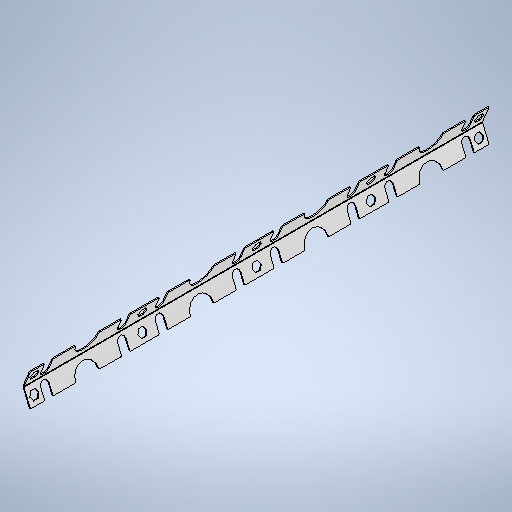
# Autodesk Inventor part: DMF 01 17 опора крышки v2.1
Saved by Autodesk Inventor 2026.2 (Build 302298010, 298A)
## iProperties
Created: 2024-04-30
Part Number: DMF 01 17 опора крышки v2.1
Material: Stainless Steel AISI 304
Document SubType Name: Sheet Metal
Designer: pokla
Density: 8 g/cm^3
Appearance: Chrome - Satin
Sheet Metal Rule: Default
Flat Pattern Width: 7.47819 cm
Flat Pattern Length: 98.3 cm
Flat Pattern Area: 735.107 cm^2
Sheet Metal Width: 74,782 mm
Sheet Metal Length: 983,000 mm
Sheet Metal Area: 73510,654 mm^2
Stock Number: Барабан_Полка_Крышки
Author: pokla
Autodesk Inventor part; units mm, degrees
ref_plane "YZ Plane" through (0, 0, 0) normal (1, 0, 0) x (0, 1, 0)
ref_plane "XZ Plane" through (0, 0, 0) normal (0, 1, 0) x (-1, 0, 0)
ref_plane "XY Plane" through (0, 0, 0) normal (0, 0, 1) x (1, 0, 0)
sketch "Sketch4" plane through (0, 0, 0) normal (0, 0, 1) x (1, 0, 0)
  line L0 (-196.316601, 196.316601) -> (0, 277.633599) construction
  line L1 (0, 277.633599) -> (196.316601, 196.316601) construction
  line L2 (196.316601, 196.316601) -> (277.633599, 0) construction
  line L3 (277.633599, 0) -> (196.316601, -196.316601) construction
  line L4 (196.316601, -196.316601) -> (0, -277.633599) construction
  line L5 (0, -277.633599) -> (-196.316601, -196.316601) construction
  line L6 (-196.316601, -196.316601) -> (-277.633599, 0) construction
  line L7 (-277.633599, 0) -> (-196.316601, 196.316601) construction
  line L8 (-276.999549, 1.530734) -> (-263.123447, 35.030606)
  line L9 (-276.999549, -1.530734) -> (-263.123447, -35.030606)
  arc A0 (-276.999549, 1.530734) -> (-276.999549, -1.530734) centre (-273.304031, 0) ccw
  point P0 (0, 0)
  point P1 (0, 0)
  point P2 (0, 0)
  dimension "d16" = 513
  dimension "d23" = 36.26
  dimension "d24" = 4
  measures "d16" distance between parallel lines of L7 L3
  measures "d23" distance of L8.start L8.end
  measures "d24" radius of A0
contour flange "Contour Flange1" sketch "Sketch4" thickness 2 bend radius 2 width 983 along (0, 0, -1) mid plane no both sides no wall seen from (-270.061498, 18.28067, 0) lies toward (0.9238795, -0.3826834, 0) curves L8 A0 L9
bend "Bend2"
corner "Corner2"
sketch "Эскиз14" plane through (-276.999549, 1.530734, -983) normal (-0.9238795, 0.3826834, 0) x (0, 0, 1)
  line L0 (0, 36.26) -> (0, 0) projected
  line L1 (983, 36.26) -> (0, 36.26) projected
  line L2 (98, 36.26) -> (98, 35.26)
  arc A0 (98, 35.26) -> (148, 35.26) centre (123, 35.26) ccw
  line L3 (148, 35.26) -> (148, 36.26)
  line L4 (40.5, 24.26) -> (205.5, 24.26) construction
  line L5 (205.5, 44.26) -> (205.5, 14.26) construction
  line L6 (196.5, 44.26) -> (196.5, 14.26)
  line L7 (214.5, 14.26) -> (214.5, 44.26)
  arc A1 (214.5, 44.26) -> (196.5, 44.26) centre (205.5, 44.26) ccw
  arc A2 (196.5, 14.26) -> (214.5, 14.26) centre (205.5, 14.26) ccw
  line L8 (123, 24.26) -> (123, 35.26) construction
  line L9 (40.5, 44.26) -> (40.5, 14.26) construction
  line L10 (31.5, 44.26) -> (31.5, 14.26)
  line L11 (49.5, 14.26) -> (49.5, 44.26)
  arc A3 (49.5, 44.26) -> (31.5, 44.26) centre (40.5, 44.26) ccw
  arc A4 (31.5, 14.26) -> (49.5, 14.26) centre (40.5, 14.26) ccw
  point P0 (205.5, 29.26)
  point P1 (40.5, 20.838326)
  point P2 (40.5, 29.26)
  point P3 (48.946898, 36.26)
  point P4 (36.053102, 36.26)
  point P5 (201.053102, 36.26)
  point P6 (213.946898, 36.26)
  point P7 (31.5, 36.26)
  point P8 (49.5, 36.26)
  point P9 (214.5, 36.26)
  point P10 (196.5, 36.26)
  dimension "d102" = 12
  dimension "d103" = 165
  dimension "d135" = 1
  dimension "d136" = 25
  dimension "d137" = 18
  dimension "d139" = 10
  dimension "d140" = 20
  dimension "d141" = 18
  dimension "d150" = 98
  constraints: 24 end point, 10 point on circle, 10 tangent, 5 centre point, 5 point on line, 4 horizontal alignment, 3 midpoint, 3 vertical, 2 parallel, 2 perpendicular, 1 horizontal, 1 vertical alignment
  measures "d102" distance from line of L1 L4.start
  measures "d103" distance of L4.end L4.start
  measures "d135" distance from line of L1 L8.end
  measures "d136" radius of A0
  measures "d137" diameter of A2
  measures "d139" distance from line of L5.end L4
  measures "d140" distance from line of L4 L5.start
  measures "d141" diameter of A4
  measures "d150" distance between parallel lines of L0 L2
extrude "Выдавливание8" cut sketch "Эскиз14" against normal through all contours L3 A0 L2 L1 | L7 A2 L6 L1 | L11 A4 L10 L1
sketch "Sketch6" plane through (-276.999549, 1.530734, 0) normal (-0.9238795, 0.3826834, 0) x (0.3826834, 0.9238795, 0)
  circle A0 centre (19.22, 15) radius 5.5 construction
  circle A1 centre (19.22, 968) radius 5.5 construction
  line L0 (0, 0) -> (0, 983)
  line L1 (36.26, 983) -> (0, 983)
  line L2 (36.26, 0) -> (0, 0)
  line L3 (27.62, 963.150258) -> (19.22, 958.300515)
  line L4 (19.22, 958.300515) -> (10.82, 963.150258)
  line L5 (10.82, 963.150258) -> (10.82, 972.849742)
  line L6 (10.82, 972.849742) -> (19.22, 977.699485)
  line L7 (19.22, 977.699485) -> (27.62, 972.849742)
  line L8 (27.62, 972.849742) -> (27.62, 963.150258)
  line L9 (27.62, 10.150258) -> (19.22, 5.300515)
  line L10 (19.22, 5.300515) -> (10.82, 10.150258)
  line L11 (10.82, 10.150258) -> (10.82, 19.849742)
  line L12 (10.82, 19.849742) -> (19.22, 24.699485)
  line L13 (19.22, 24.699485) -> (27.62, 19.849742)
  line L14 (27.62, 19.849742) -> (27.62, 10.150258)
  circle A2 centre (19.22, 736.5) radius 5.5 construction
  line L15 (27.62, 731.650258) -> (19.22, 726.800515)
  line L16 (19.22, 726.800515) -> (10.82, 731.650258)
  line L17 (10.82, 731.650258) -> (10.82, 741.349742)
  line L18 (10.82, 741.349742) -> (19.22, 746.199485)
  line L19 (19.22, 746.199485) -> (27.62, 741.349742)
  line L20 (27.62, 741.349742) -> (27.62, 731.650258)
  circle A3 centre (19.22, 491.5) radius 5.5 construction
  line L21 (27.62, 486.650258) -> (19.22, 481.800515)
  line L22 (19.22, 481.800515) -> (10.82, 486.650258)
  line L23 (10.82, 486.650258) -> (10.82, 496.349742)
  line L24 (10.82, 496.349742) -> (19.22, 501.199485)
  line L25 (19.22, 501.199485) -> (27.62, 496.349742)
  line L26 (27.62, 496.349742) -> (27.62, 486.650258)
  circle A4 centre (19.22, 246.5) radius 5.5 construction
  line L27 (27.62, 241.650258) -> (19.22, 236.800515)
  line L28 (19.22, 236.800515) -> (10.82, 241.650258)
  line L29 (10.82, 241.650258) -> (10.82, 251.349742)
  line L30 (10.82, 251.349742) -> (19.22, 256.199485)
  line L31 (19.22, 256.199485) -> (27.62, 251.349742)
  line L32 (27.62, 251.349742) -> (27.62, 241.650258)
  line L33 (36.26, 0) -> (36.26, 983)
  point P0 (104.588924, 0)
  dimension "d36" = 11
  dimension "d41" = 11
  dimension "d93" = 19.22
  dimension "d95" = 19.22
  dimension "d98" = 16.8
  dimension "d99" = 16.8
  dimension "d120" = 15
  dimension "d121" = 15
  dimension "d122" = 11
  dimension "d123" = 16.8
  dimension "d125" = 11
  dimension "d126" = 16.8
  dimension "d128" = 11
  dimension "d129" = 16.8
  dimension "d131" = 231.5
  dimension "d132" = 245
  dimension "d133" = 245
  dimension "d152" = 231.5
  constraints: 60 end point, 5 centre point, 5 coincident, 5 parallel, 3 vertical alignment, 65 other
  measures "d36" diameter of A0
  measures "d41" diameter of A1
  measures "d93" distance from line of L0 A0.centre
  measures "d95" distance from line of L0 A1.centre
  measures "d98" distance between parallel lines of L6 L3
  measures "d99" distance between parallel lines of L12 L9
  measures "d120" distance from line of L1 A1.centre
  measures "d121" distance from line of L2 point (19.22, 15)
  measures "d122" diameter of A2
  measures "d123" distance between parallel lines of L18 L15
  measures "d125" diameter of A3
  measures "d126" distance between parallel lines of L24 L21
  measures "d128" diameter of A4
  measures "d129" distance between parallel lines of L30 L27
  measures "d131" distance of A2.centre point (19.22, 968)
  measures "d132" distance of A3.centre A2.centre
  measures "d133" distance of A4.centre A3.centre
  measures "d152" distance of A4.centre A0.centre
extrude "Extrusion1" cut sketch "Sketch6" against normal up to surface (2 mm away) contours L3 L4 L5 L6 L7 L8 | L9 L10 L11 L12 L13 L14 | L15 L16 L17 L18 L19 L20 | L21 L22 L23 L24 L25 L26 | L27 L28 L29 L30 L31 L32
pattern_linear "Rectangular Pattern9" count 4 spacing 246 along (0, 0, 1) of "Выдавливание8"
mirror "Mirror4" about plane through (0, 0, 0) normal (0, 1, 0) of "Выдавливание8", "Extrusion1"
mirror "Mirror5" about plane through (0, 0, 0) normal (0, 1, 0) of "Выдавливание8", "Rectangular Pattern9", "Extrusion1"
fillet "Corner Round2" radius 2 48 edges at (-262.1996, 34.6479, -951.5) (-262.1996, 34.6479, -933.5) (-262.1996, -34.6479, -933.5) (-262.1996, -34.6479, -951.5) (-262.1996, -34.6479, -786.5) (-262.1996, -34.6479, -768.5) (-262.1996, 34.6479, -768.5) (-262.1996, 34.6479, -786.5) (-262.1996, 34.6479, -705.5) (-262.1996, 34.6479, -687.5) (-262.1996, -34.6479, -687.5) (-262.1996, -34.6479, -705.5) (-262.1996, -34.6479, -522.5) (-262.1996, 34.6479, -522.5) (-262.1996, -34.6479, -540.5) (-262.1996, 34.6479, -540.5) (-262.1996, 34.6479, -441.5) (-262.1996, 34.6479, -459.5) (-262.1996, -34.6479, -459.5) (-262.1996, -34.6479, -441.5) (-262.1996, 34.6479, -276.5) (-262.1996, 34.6479, -294.5) (-262.1996, -34.6479, -276.5) (-262.1996, -34.6479, -294.5) (-262.1996, 34.6479, -213.5) (-262.1996, 34.6479, -195.5) (-262.1996, -34.6479, -213.5) (-262.1996, -34.6479, -195.5) (-262.1996, 34.6479, -30.5) (-262.1996, 34.6479, -48.5) (-262.1996, -34.6479, -30.5) (-262.1996, -34.6479, -48.5) (-262.1996, 34.6479, -147) (-262.1996, 34.6479, -97) (-262.1996, -34.6479, -147) (-262.1996, -34.6479, -97) (-262.1996, 34.6479, -393) (-262.1996, 34.6479, -343) (-262.1996, -34.6479, -343) (-262.1996, -34.6479, -393) (-262.1996, -34.6479, -589) (-262.1996, -34.6479, -639) (-262.1996, 34.6479, -639) (-262.1996, 34.6479, -589) (-262.1996, 34.6479, -835) (-262.1996, 34.6479, -885) (-262.1996, -34.6479, -835) (-262.1996, -34.6479, -885)
equation "\"d16\" = Барабан_размер_по_плоскостям - Thickness"
equation "\"d24\" = BendRadius + Thickness"
equation "\"d41\" = d36"
equation "\"d95\" = d93"
equation "\"d99\" = d98"
equation "\"d122\" = d124"
equation "\"d125\" = d127"
equation "\"d128\" = d130"
equation "\"d25\" = Thickness"
equation "\"d26\" = BendReliefWidth"
equation "\"d27\" = BendReliefDepth"
equation "\"d28\" = MinimumRemnant"
equation "\"d29\" = TransitionRadius"
equation "\"d31\" = BendRadius"
equation "\"d33\" = CornerReliefSize"
equation "\"d34\" = GapSize"
equation "\"d35\" = JacobiRadiusSize"
equation "\"BendRadius\" = Thickness"
equation "\"BendReliefWidth\" = Thickness"
equation "\"BendReliefDepth\" = 0.5 * Thickness"
equation "\"CornerReliefSize\" = 4 * Thickness"
equation "\"MinimumRemnant\" = 2 * Thickness"
equation "\"TransitionRadius\" = BendRadius"
equation "\"JacobiRadiusSize\" = BendRadius"
equation "\"GapSize\" = Thickness"
equation "\"Барабан_размер_по_плоскостям\" = 515"
equation "\"Thickness\" = 2"
equation "\"d124\" = 11"
equation "\"d127\" = 11"
equation "\"d130\" = 11"
body "Solid2"
